Autodesk Inventor part; units mm, degrees
(part 2 of 3)
sketch "Sketch2" plane through (2, 0, 0) normal (1, 0, 0) x (0, 0, -1)
  line L0 (22.4898, 96.0981) -> (22.4898, 576.0981) projected
  line L1 (22.4898, 576.0981) -> (-367.5102, 576.0981) projected
  line L2 (-367.5102, 576.0981) -> (-367.5102, 96.0981) projected
  line L3 (-367.5102, 96.0981) -> (22.4898, 96.0981) projected
  circle A0 centre (-42.5102, 103.5981) radius 1.75 projected
  circle A1 centre (-302.5102, 568.5981) radius 1.75 projected
  circle A2 centre (-42.5102, 568.5981) radius 1.75 projected
  circle A3 centre (-360.0102, 161.0981) radius 1.75 projected
  circle A4 centre (-360.0102, 511.0981) radius 1.75 projected
  circle A5 centre (14.9898, 161.0981) radius 1.75 projected
  circle A6 centre (14.9898, 511.0981) radius 1.75 projected
  circle A7 centre (-172.5102, 568.5981) radius 1.75 projected
  circle A8 centre (-302.5102, 103.5981) radius 1.75 projected
  line L4 (2.265, 163.0981) -> (-3.5085, 163.0981) projected
  line L5 (-3.5085, 163.0981) -> (-6.3952, 168.0981) projected
  line L6 (-6.3952, 168.0981) -> (-3.5085, 173.0981) projected
  line L7 (-3.5085, 173.0981) -> (2.265, 173.0981) projected
  line L8 (2.265, 173.0981) -> (5.1518, 168.0981) projected
  line L9 (5.1518, 168.0981) -> (2.265, 163.0981) projected
  line L10 (-23.735, 143.0981) -> (-20.8482, 138.0981) projected
  line L11 (-20.8482, 138.0981) -> (-23.735, 133.0981) projected
  line L12 (-23.735, 133.0981) -> (-29.5085, 133.0981) projected
  line L13 (-29.5085, 133.0981) -> (-32.3952, 138.0981) projected
  line L14 (-32.3952, 138.0981) -> (-29.5085, 143.0981) projected
  line L15 (-29.5085, 143.0981) -> (-23.735, 143.0981) projected
  line L16 (-45.3856, 160.5981) -> (-42.4988, 165.5981) projected
  line L17 (-42.4988, 165.5981) -> (-36.7253, 165.5981) projected
  line L18 (-36.7253, 165.5981) -> (-33.8386, 160.5981) projected
  line L19 (-33.8386, 160.5981) -> (-36.7253, 155.5981) projected
  line L20 (-36.7253, 155.5981) -> (-42.4988, 155.5981) projected
  line L21 (-42.4988, 155.5981) -> (-45.3856, 160.5981) projected
  line L22 (-55.5085, 128.0981) -> (-49.735, 128.0981) projected
  line L23 (-49.735, 128.0981) -> (-46.8482, 123.0981) projected
  line L24 (-46.8482, 123.0981) -> (-49.735, 118.0981) projected
  line L25 (-49.735, 118.0981) -> (-55.5085, 118.0981) projected
  line L26 (-55.5085, 118.0981) -> (-58.3952, 123.0981) projected
  line L27 (-58.3952, 123.0981) -> (-55.5085, 128.0981) projected
  line L28 (-72.8482, 168.0981) -> (-75.735, 163.0981) projected
  line L29 (-75.735, 163.0981) -> (-81.5085, 163.0981) projected
  line L30 (-81.5085, 163.0981) -> (-84.3952, 168.0981) projected
  line L31 (-84.3952, 168.0981) -> (-81.5085, 173.0981) projected
  line L32 (-81.5085, 173.0981) -> (-75.735, 173.0981) projected
  line L33 (-75.735, 173.0981) -> (-72.8482, 168.0981) projected
  line L34 (-97.3856, 130.5981) -> (-94.4988, 135.5981) projected
  line L35 (-94.4988, 135.5981) -> (-88.7253, 135.5981) projected
  line L36 (-88.7253, 135.5981) -> (-85.8386, 130.5981) projected
  line L37 (-85.8386, 130.5981) -> (-88.7253, 125.5981) projected
  line L38 (-88.7253, 125.5981) -> (-94.4988, 125.5981) projected
  line L39 (-94.4988, 125.5981) -> (-97.3856, 130.5981) projected
  line L40 (-107.5085, 158.0981) -> (-101.735, 158.0981) projected
  line L41 (-101.735, 158.0981) -> (-98.8482, 153.0981) projected
  line L42 (-98.8482, 153.0981) -> (-101.735, 148.0981) projected
  line L43 (-101.735, 148.0981) -> (-107.5085, 148.0981) projected
  line L44 (-107.5085, 148.0981) -> (-110.3952, 153.0981) projected
  line L45 (-110.3952, 153.0981) -> (-107.5085, 158.0981) projected
  line L46 (-120.4988, 140.5981) -> (-123.3856, 145.5981) projected
  line L47 (-123.3856, 145.5981) -> (-120.4988, 150.5981) projected
  line L48 (-120.4988, 150.5981) -> (-114.7253, 150.5981) projected
  line L49 (-114.7253, 150.5981) -> (-111.8386, 145.5981) projected
  line L50 (-111.8386, 145.5981) -> (-114.7253, 140.5981) projected
  line L51 (-114.7253, 140.5981) -> (-120.4988, 140.5981) projected
  line L52 (-127.735, 143.0981) -> (-124.8482, 138.0981) projected
  line L53 (-124.8482, 138.0981) -> (-127.735, 133.0981) projected
  line L54 (-127.735, 133.0981) -> (-133.5085, 133.0981) projected
  line L55 (-133.5085, 133.0981) -> (-136.3952, 138.0981) projected
  line L56 (-136.3952, 138.0981) -> (-133.5085, 143.0981) projected
  line L57 (-133.5085, 143.0981) -> (-127.735, 143.0981) projected
  line L58 (-153.735, 143.0981) -> (-150.8482, 138.0981) projected
  line L59 (-150.8482, 138.0981) -> (-153.735, 133.0981) projected
  line L60 (-153.735, 133.0981) -> (-159.5085, 133.0981) projected
  line L61 (-159.5085, 133.0981) -> (-162.3952, 138.0981) projected
  line L62 (-162.3952, 138.0981) -> (-159.5085, 143.0981) projected
  line L63 (-159.5085, 143.0981) -> (-153.735, 143.0981) projected
  line L64 (-159.5085, 158.0981) -> (-153.735, 158.0981) projected
  line L65 (-153.735, 158.0981) -> (-150.8482, 153.0981) projected
  line L66 (-150.8482, 153.0981) -> (-153.735, 148.0981) projected
  line L67 (-153.735, 148.0981) -> (-159.5085, 148.0981) projected
  line L68 (-159.5085, 148.0981) -> (-162.3952, 153.0981) projected
  line L69 (-162.3952, 153.0981) -> (-159.5085, 158.0981) projected
  line L70 (-176.8482, 168.0981) -> (-179.735, 163.0981) projected
  line L71 (-179.735, 163.0981) -> (-185.5085, 163.0981) projected
  line L72 (-185.5085, 163.0981) -> (-188.3952, 168.0981) projected
  line L73 (-188.3952, 168.0981) -> (-185.5085, 173.0981) projected
  line L74 (-185.5085, 173.0981) -> (-179.735, 173.0981) projected
  line L75 (-179.735, 173.0981) -> (-176.8482, 168.0981) projected
  line L76 (-201.3856, 130.5981) -> (-198.4988, 135.5981) projected
  line L77 (-198.4988, 135.5981) -> (-192.7253, 135.5981) projected
  line L78 (-192.7253, 135.5981) -> (-189.8386, 130.5981) projected
  line L79 (-189.8386, 130.5981) -> (-192.7253, 125.5981) projected
  line L80 (-192.7253, 125.5981) -> (-198.4988, 125.5981) projected
  line L81 (-198.4988, 125.5981) -> (-201.3856, 130.5981) projected
  line L82 (-211.5085, 158.0981) -> (-205.735, 158.0981) projected
  line L83 (-205.735, 158.0981) -> (-202.8482, 153.0981) projected
  line L84 (-202.8482, 153.0981) -> (-205.735, 148.0981) projected
  line L85 (-205.735, 148.0981) -> (-211.5085, 148.0981) projected
  line L86 (-211.5085, 148.0981) -> (-214.3952, 153.0981) projected
  line L87 (-214.3952, 153.0981) -> (-211.5085, 158.0981) projected
  line L88 (-224.4988, 140.5981) -> (-227.3856, 145.5981) projected
  line L89 (-227.3856, 145.5981) -> (-224.4988, 150.5981) projected
  line L90 (-224.4988, 150.5981) -> (-218.7253, 150.5981) projected
  line L91 (-218.7253, 150.5981) -> (-215.8386, 145.5981) projected
  line L92 (-215.8386, 145.5981) -> (-218.7253, 140.5981) projected
  line L93 (-218.7253, 140.5981) -> (-224.4988, 140.5981) projected
  line L94 (-231.735, 143.0981) -> (-228.8482, 138.0981) projected
  line L95 (-228.8482, 138.0981) -> (-231.735, 133.0981) projected
  line L96 (-231.735, 133.0981) -> (-237.5085, 133.0981) projected
  line L97 (-237.5085, 133.0981) -> (-240.3952, 138.0981) projected
  line L98 (-240.3952, 138.0981) -> (-237.5085, 143.0981) projected
  line L99 (-237.5085, 143.0981) -> (-231.735, 143.0981) projected
  line L100 (-253.3856, 160.5981) -> (-250.4988, 165.5981) projected
  line L101 (-250.4988, 165.5981) -> (-244.7253, 165.5981) projected
  line L102 (-244.7253, 165.5981) -> (-241.8386, 160.5981) projected
  line L103 (-241.8386, 160.5981) -> (-244.7253, 155.5981) projected
  line L104 (-244.7253, 155.5981) -> (-250.4988, 155.5981) projected
  line L105 (-250.4988, 155.5981) -> (-253.3856, 160.5981) projected
  line L106 (-263.5085, 128.0981) -> (-257.735, 128.0981) projected
  line L107 (-257.735, 128.0981) -> (-254.8482, 123.0981) projected
  line L108 (-254.8482, 123.0981) -> (-257.735, 118.0981) projected
  line L109 (-257.735, 118.0981) -> (-263.5085, 118.0981) projected
  line L110 (-263.5085, 118.0981) -> (-266.3952, 123.0981) projected
  line L111 (-266.3952, 123.0981) -> (-263.5085, 128.0981) projected
  line L112 (-315.5085, 128.0981) -> (-309.735, 128.0981) projected
  line L113 (-309.735, 128.0981) -> (-306.8482, 123.0981) projected
  line L114 (-306.8482, 123.0981) -> (-309.735, 118.0981) projected
  line L115 (-309.735, 118.0981) -> (-315.5085, 118.0981) projected
  line L116 (-315.5085, 118.0981) -> (-318.3952, 123.0981) projected
  line L117 (-318.3952, 123.0981) -> (-315.5085, 128.0981) projected
  line L118 (-341.5085, 158.0981) -> (-335.735, 158.0981) projected
  line L119 (-335.735, 158.0981) -> (-332.8482, 153.0981) projected
  line L120 (-332.8482, 153.0981) -> (-335.735, 148.0981) projected
  line L121 (-335.735, 148.0981) -> (-341.5085, 148.0981) projected
  line L122 (-341.5085, 148.0981) -> (-344.3952, 153.0981) projected
  line L123 (-344.3952, 153.0981) -> (-341.5085, 158.0981) projected
  line L124 (-280.8482, 168.0981) -> (-283.735, 163.0981) projected
  line L125 (-283.735, 163.0981) -> (-289.5085, 163.0981) projected
  line L126 (-289.5085, 163.0981) -> (-292.3952, 168.0981) projected
  line L127 (-292.3952, 168.0981) -> (-289.5085, 173.0981) projected
  line L128 (-289.5085, 173.0981) -> (-283.735, 173.0981) projected
  line L129 (-283.735, 173.0981) -> (-280.8482, 168.0981) projected
  line L130 (-283.735, 143.0981) -> (-280.8482, 138.0981) projected
  line L131 (-280.8482, 138.0981) -> (-283.735, 133.0981) projected
  line L132 (-283.735, 133.0981) -> (-289.5085, 133.0981) projected
  line L133 (-289.5085, 133.0981) -> (-292.3952, 138.0981) projected
  line L134 (-292.3952, 138.0981) -> (-289.5085, 143.0981) projected
  line L135 (-289.5085, 143.0981) -> (-283.735, 143.0981) projected
  line L136 (-309.735, 143.0981) -> (-306.8482, 138.0981) projected
  line L137 (-306.8482, 138.0981) -> (-309.735, 133.0981) projected
  line L138 (-309.735, 133.0981) -> (-315.5085, 133.0981) projected
  line L139 (-315.5085, 133.0981) -> (-318.3952, 138.0981) projected
  line L140 (-318.3952, 138.0981) -> (-315.5085, 143.0981) projected
  line L141 (-315.5085, 143.0981) -> (-309.735, 143.0981) projected
  line L142 (-3.5085, 128.0981) -> (2.265, 128.0981) projected
  line L143 (2.265, 128.0981) -> (5.1518, 123.0981) projected
  line L144 (5.1518, 123.0981) -> (2.265, 118.0981) projected
  line L145 (2.265, 118.0981) -> (-3.5085, 118.0981) projected
  line L146 (-3.5085, 118.0981) -> (-6.3952, 123.0981) projected
  line L147 (-6.3952, 123.0981) -> (-3.5085, 128.0981) projected
  line L148 (-10.7253, 140.5981) -> (-16.4988, 140.5981) projected
  line L149 (-16.4988, 140.5981) -> (-19.3856, 145.5981) projected
  line L150 (-19.3856, 145.5981) -> (-16.4988, 150.5981) projected
  line L151 (-16.4988, 150.5981) -> (-10.7253, 150.5981) projected
  line L152 (-10.7253, 150.5981) -> (-7.8386, 145.5981) projected
  line L153 (-7.8386, 145.5981) -> (-10.7253, 140.5981) projected
  line L154 (-328.4988, 140.5981) -> (-331.3856, 145.5981) projected
  line L155 (-331.3856, 145.5981) -> (-328.4988, 150.5981) projected
  line L156 (-328.4988, 150.5981) -> (-322.7253, 150.5981) projected
  line L157 (-322.7253, 150.5981) -> (-319.8386, 145.5981) projected
  line L158 (-319.8386, 145.5981) -> (-322.7253, 140.5981) projected
  line L159 (-322.7253, 140.5981) -> (-328.4988, 140.5981) projected
  line L160 (-302.4988, 140.5981) -> (-305.3856, 145.5981) projected
  line L161 (-305.3856, 145.5981) -> (-302.4988, 150.5981) projected
  line L162 (-302.4988, 150.5981) -> (-296.7253, 150.5981) projected
  line L163 (-296.7253, 150.5981) -> (-293.8386, 145.5981) projected
  line L164 (-293.8386, 145.5981) -> (-296.7253, 140.5981) projected
  line L165 (-296.7253, 140.5981) -> (-302.4988, 140.5981) projected
  line L166 (-279.3856, 160.5981) -> (-276.4988, 165.5981) projected
  line L167 (-276.4988, 165.5981) -> (-270.7253, 165.5981) projected
  line L168 (-270.7253, 165.5981) -> (-267.8386, 160.5981) projected
  line L169 (-267.8386, 160.5981) -> (-270.7253, 155.5981) projected
  line L170 (-270.7253, 155.5981) -> (-276.4988, 155.5981) projected
  line L171 (-276.4988, 155.5981) -> (-279.3856, 160.5981) projected
  line L172 (-332.8482, 168.0981) -> (-335.735, 163.0981) projected
  line L173 (-335.735, 163.0981) -> (-341.5085, 163.0981) projected
  line L174 (-341.5085, 163.0981) -> (-344.3952, 168.0981) projected
  line L175 (-344.3952, 168.0981) -> (-341.5085, 173.0981) projected
  line L176 (-341.5085, 173.0981) -> (-335.735, 173.0981) projected
  line L177 (-335.735, 173.0981) -> (-332.8482, 168.0981) projected
  line L178 (-331.3856, 130.5981) -> (-328.4988, 135.5981) projected
  line L179 (-328.4988, 135.5981) -> (-322.7253, 135.5981) projected
  line L180 (-322.7253, 135.5981) -> (-319.8386, 130.5981) projected
  line L181 (-319.8386, 130.5981) -> (-322.7253, 125.5981) projected
  line L182 (-322.7253, 125.5981) -> (-328.4988, 125.5981) projected
  line L183 (-328.4988, 125.5981) -> (-331.3856, 130.5981) projected
  line L184 (-279.3856, 130.5981) -> (-276.4988, 135.5981) projected
  line L185 (-276.4988, 135.5981) -> (-270.7253, 135.5981) projected
  line L186 (-270.7253, 135.5981) -> (-267.8386, 130.5981) projected
  line L187 (-267.8386, 130.5981) -> (-270.7253, 125.5981) projected
  line L188 (-270.7253, 125.5981) -> (-276.4988, 125.5981) projected
  line L189 (-276.4988, 125.5981) -> (-279.3856, 130.5981) projected
  line L190 (-254.8482, 168.0981) -> (-257.735, 163.0981) projected
  line L191 (-257.735, 163.0981) -> (-263.5085, 163.0981) projected
  line L192 (-263.5085, 163.0981) -> (-266.3952, 168.0981) projected
  line L193 (-266.3952, 168.0981) -> (-263.5085, 173.0981) projected
  line L194 (-263.5085, 173.0981) -> (-257.735, 173.0981) projected
  line L195 (-257.735, 173.0981) -> (-254.8482, 168.0981) projected
  line L196 (-237.5085, 128.0981) -> (-231.735, 128.0981) projected
  line L197 (-231.735, 128.0981) -> (-228.8482, 123.0981) projected
  line L198 (-228.8482, 123.0981) -> (-231.735, 118.0981) projected
  line L199 (-231.735, 118.0981) -> (-237.5085, 118.0981) projected
  line L200 (-237.5085, 118.0981) -> (-240.3952, 123.0981) projected
  line L201 (-240.3952, 123.0981) -> (-237.5085, 128.0981) projected
  line L202 (-227.3856, 160.5981) -> (-224.4988, 165.5981) projected
  line L203 (-224.4988, 165.5981) -> (-218.7253, 165.5981) projected
  line L204 (-218.7253, 165.5981) -> (-215.8386, 160.5981) projected
  line L205 (-215.8386, 160.5981) -> (-218.7253, 155.5981) projected
  line L206 (-218.7253, 155.5981) -> (-224.4988, 155.5981) projected
  line L207 (-224.4988, 155.5981) -> (-227.3856, 160.5981) projected
  line L208 (-205.735, 143.0981) -> (-202.8482, 138.0981) projected
  line L209 (-202.8482, 138.0981) -> (-205.735, 133.0981) projected
  line L210 (-205.735, 133.0981) -> (-211.5085, 133.0981) projected
  line L211 (-211.5085, 133.0981) -> (-214.3952, 138.0981) projected
  line L212 (-214.3952, 138.0981) -> (-211.5085, 143.0981) projected
  line L213 (-211.5085, 143.0981) -> (-205.735, 143.0981) projected
  line L214 (-198.4988, 140.5981) -> (-201.3856, 145.5981) projected
  line L215 (-201.3856, 145.5981) -> (-198.4988, 150.5981) projected
  line L216 (-198.4988, 150.5981) -> (-192.7253, 150.5981) projected
  line L217 (-192.7253, 150.5981) -> (-189.8386, 145.5981) projected
  line L218 (-189.8386, 145.5981) -> (-192.7253, 140.5981) projected
  line L219 (-192.7253, 140.5981) -> (-198.4988, 140.5981) projected
  line L220 (-185.5085, 158.0981) -> (-179.735, 158.0981) projected
  line L221 (-179.735, 158.0981) -> (-176.8482, 153.0981) projected
  line L222 (-176.8482, 153.0981) -> (-179.735, 148.0981) projected
  line L223 (-179.735, 148.0981) -> (-185.5085, 148.0981) projected
  line L224 (-185.5085, 148.0981) -> (-188.3952, 153.0981) projected
  line L225 (-188.3952, 153.0981) -> (-185.5085, 158.0981) projected
  line L226 (-175.3856, 130.5981) -> (-172.4988, 135.5981) projected
  line L227 (-172.4988, 135.5981) -> (-166.7253, 135.5981) projected
  line L228 (-166.7253, 135.5981) -> (-163.8386, 130.5981) projected
  line L229 (-163.8386, 130.5981) -> (-166.7253, 125.5981) projected
  line L230 (-166.7253, 125.5981) -> (-172.4988, 125.5981) projected
  line L231 (-172.4988, 125.5981) -> (-175.3856, 130.5981) projected
  line L232 (-146.4988, 140.5981) -> (-149.3856, 145.5981) projected
  line L233 (-149.3856, 145.5981) -> (-146.4988, 150.5981) projected
  line L234 (-146.4988, 150.5981) -> (-140.7253, 150.5981) projected
  line L235 (-140.7253, 150.5981) -> (-137.8386, 145.5981) projected
  line L236 (-137.8386, 145.5981) -> (-140.7253, 140.5981) projected
  line L237 (-140.7253, 140.5981) -> (-146.4988, 140.5981) projected
  line L238 (-133.5085, 128.0981) -> (-127.735, 128.0981) projected
  line L239 (-127.735, 128.0981) -> (-124.8482, 123.0981) projected
  line L240 (-124.8482, 123.0981) -> (-127.735, 118.0981) projected
  line L241 (-127.735, 118.0981) -> (-133.5085, 118.0981) projected
  line L242 (-133.5085, 118.0981) -> (-136.3952, 123.0981) projected
  line L243 (-136.3952, 123.0981) -> (-133.5085, 128.0981) projected
  line L244 (-123.3856, 160.5981) -> (-120.4988, 165.5981) projected
  line L245 (-120.4988, 165.5981) -> (-114.7253, 165.5981) projected
  line L246 (-114.7253, 165.5981) -> (-111.8386, 160.5981) projected
  line L247 (-111.8386, 160.5981) -> (-114.7253, 155.5981) projected
  line L248 (-114.7253, 155.5981) -> (-120.4988, 155.5981) projected
  line L249 (-120.4988, 155.5981) -> (-123.3856, 160.5981) projected
  line L250 (-101.735, 143.0981) -> (-98.8482, 138.0981) projected
  line L251 (-98.8482, 138.0981) -> (-101.735, 133.0981) projected
  line L252 (-101.735, 133.0981) -> (-107.5085, 133.0981) projected
  line L253 (-107.5085, 133.0981) -> (-110.3952, 138.0981) projected
  line L254 (-110.3952, 138.0981) -> (-107.5085, 143.0981) projected
  line L255 (-107.5085, 143.0981) -> (-101.735, 143.0981) projected
  line L256 (-94.4988, 140.5981) -> (-97.3856, 145.5981) projected
  line L257 (-97.3856, 145.5981) -> (-94.4988, 150.5981) projected
  line L258 (-94.4988, 150.5981) -> (-88.7253, 150.5981) projected
  line L259 (-88.7253, 150.5981) -> (-85.8386, 145.5981) projected
  line L260 (-85.8386, 145.5981) -> (-88.7253, 140.5981) projected
  line L261 (-88.7253, 140.5981) -> (-94.4988, 140.5981) projected
  line L262 (-81.5085, 158.0981) -> (-75.735, 158.0981) projected
  line L263 (-75.735, 158.0981) -> (-72.8482, 153.0981) projected
  line L264 (-72.8482, 153.0981) -> (-75.735, 148.0981) projected
  line L265 (-75.735, 148.0981) -> (-81.5085, 148.0981) projected
  line L266 (-81.5085, 148.0981) -> (-84.3952, 153.0981) projected
  line L267 (-84.3952, 153.0981) -> (-81.5085, 158.0981) projected
  line L268 (-71.3856, 130.5981) -> (-68.4988, 135.5981) projected
  line L269 (-68.4988, 135.5981) -> (-62.7253, 135.5981) projected
  line L270 (-62.7253, 135.5981) -> (-59.8386, 130.5981) projected
  line L271 (-59.8386, 130.5981) -> (-62.7253, 125.5981) projected
  line L272 (-62.7253, 125.5981) -> (-68.4988, 125.5981) projected
  line L273 (-68.4988, 125.5981) -> (-71.3856, 130.5981) projected
  line L274 (-46.8482, 168.0981) -> (-49.735, 163.0981) projected
  line L275 (-49.735, 163.0981) -> (-55.5085, 163.0981) projected
  line L276 (-55.5085, 163.0981) -> (-58.3952, 168.0981) projected
  line L277 (-58.3952, 168.0981) -> (-55.5085, 173.0981) projected
  line L278 (-55.5085, 173.0981) -> (-49.735, 173.0981) projected
  line L279 (-49.735, 173.0981) -> (-46.8482, 168.0981) projected
  line L280 (-29.5085, 128.0981) -> (-23.735, 128.0981) projected
  line L281 (-23.735, 128.0981) -> (-20.8482, 123.0981) projected
  line L282 (-20.8482, 123.0981) -> (-23.735, 118.0981) projected
  line L283 (-23.735, 118.0981) -> (-29.5085, 118.0981) projected
  line L284 (-29.5085, 118.0981) -> (-32.3952, 123.0981) projected
  line L285 (-32.3952, 123.0981) -> (-29.5085, 128.0981) projected
  line L286 (-10.7253, 155.5981) -> (-16.4988, 155.5981) projected
  line L287 (-16.4988, 155.5981) -> (-19.3856, 160.5981) projected
  line L288 (-19.3856, 160.5981) -> (-16.4988, 165.5981) projected
  line L289 (-16.4988, 165.5981) -> (-10.7253, 165.5981) projected
  line L290 (-10.7253, 165.5981) -> (-7.8386, 160.5981) projected
  line L291 (-7.8386, 160.5981) -> (-10.7253, 155.5981) projected
  line L292 (-29.5085, 158.0981) -> (-23.735, 158.0981) projected
  line L293 (-23.735, 158.0981) -> (-20.8482, 153.0981) projected
  line L294 (-20.8482, 153.0981) -> (-23.735, 148.0981) projected
  line L295 (-23.735, 148.0981) -> (-29.5085, 148.0981) projected
  line L296 (-29.5085, 148.0981) -> (-32.3952, 153.0981) projected
  line L297 (-32.3952, 153.0981) -> (-29.5085, 158.0981) projected
  line L298 (-42.4988, 140.5981) -> (-45.3856, 145.5981) projected
  line L299 (-45.3856, 145.5981) -> (-42.4988, 150.5981) projected
  line L300 (-42.4988, 150.5981) -> (-36.7253, 150.5981) projected
  line L301 (-36.7253, 150.5981) -> (-33.8386, 145.5981) projected
  line L302 (-33.8386, 145.5981) -> (-36.7253, 140.5981) projected
  line L303 (-36.7253, 140.5981) -> (-42.4988, 140.5981) projected
  line L304 (-49.735, 143.0981) -> (-46.8482, 138.0981) projected
  line L305 (-46.8482, 138.0981) -> (-49.735, 133.0981) projected
  line L306 (-49.735, 133.0981) -> (-55.5085, 133.0981) projected
  line L307 (-55.5085, 133.0981) -> (-58.3952, 138.0981) projected
  line L308 (-58.3952, 138.0981) -> (-55.5085, 143.0981) projected
  line L309 (-55.5085, 143.0981) -> (-49.735, 143.0981) projected
  line L310 (-71.3856, 160.5981) -> (-68.4988, 165.5981) projected
  line L311 (-68.4988, 165.5981) -> (-62.7253, 165.5981) projected
  line L312 (-62.7253, 165.5981) -> (-59.8386, 160.5981) projected
  line L313 (-59.8386, 160.5981) -> (-62.7253, 155.5981) projected
  line L314 (-62.7253, 155.5981) -> (-68.4988, 155.5981) projected
  line L315 (-68.4988, 155.5981) -> (-71.3856, 160.5981) projected
  line L316 (-81.5085, 128.0981) -> (-75.735, 128.0981) projected
  line L317 (-75.735, 128.0981) -> (-72.8482, 123.0981) projected
  line L318 (-72.8482, 123.0981) -> (-75.735, 118.0981) projected
  line L319 (-75.735, 118.0981) -> (-81.5085, 118.0981) projected
  line L320 (-81.5085, 118.0981) -> (-84.3952, 123.0981) projected
  line L321 (-84.3952, 123.0981) -> (-81.5085, 128.0981) projected
  line L322 (-98.8482, 168.0981) -> (-101.735, 163.0981) projected
  line L323 (-101.735, 163.0981) -> (-107.5085, 163.0981) projected
  line L324 (-107.5085, 163.0981) -> (-110.3952, 168.0981) projected
  line L325 (-110.3952, 168.0981) -> (-107.5085, 173.0981) projected
  line L326 (-107.5085, 173.0981) -> (-101.735, 173.0981) projected
  line L327 (-101.735, 173.0981) -> (-98.8482, 168.0981) projected
  line L328 (-123.3856, 130.5981) -> (-120.4988, 135.5981) projected
  line L329 (-120.4988, 135.5981) -> (-114.7253, 135.5981) projected
  line L330 (-114.7253, 135.5981) -> (-111.8386, 130.5981) projected
  line L331 (-111.8386, 130.5981) -> (-114.7253, 125.5981) projected
  line L332 (-114.7253, 125.5981) -> (-120.4988, 125.5981) projected
  line L333 (-120.4988, 125.5981) -> (-123.3856, 130.5981) projected
  line L334 (-133.5085, 158.0981) -> (-127.735, 158.0981) projected
  line L335 (-127.735, 158.0981) -> (-124.8482, 153.0981) projected
  line L336 (-124.8482, 153.0981) -> (-127.735, 148.0981) projected
  line L337 (-127.735, 148.0981) -> (-133.5085, 148.0981) projected
  line L338 (-133.5085, 148.0981) -> (-136.3952, 153.0981) projected
  line L339 (-136.3952, 153.0981) -> (-133.5085, 158.0981) projected
  line L340 (-159.5085, 128.0981) -> (-153.735, 128.0981) projected
  line L341 (-153.735, 128.0981) -> (-150.8482, 123.0981) projected
  line L342 (-150.8482, 123.0981) -> (-153.735, 118.0981) projected
  line L343 (-153.735, 118.0981) -> (-159.5085, 118.0981) projected
  line L344 (-159.5085, 118.0981) -> (-162.3952, 123.0981) projected
  line L345 (-162.3952, 123.0981) -> (-159.5085, 128.0981) projected
  line L346 (-150.8482, 168.0981) -> (-153.735, 163.0981) projected
  line L347 (-153.735, 163.0981) -> (-159.5085, 163.0981) projected
  line L348 (-159.5085, 163.0981) -> (-162.3952, 168.0981) projected
  line L349 (-162.3952, 168.0981) -> (-159.5085, 173.0981) projected
  line L350 (-159.5085, 173.0981) -> (-153.735, 173.0981) projected
  line L351 (-153.735, 173.0981) -> (-150.8482, 168.0981) projected
  line L352 (-175.3856, 160.5981) -> (-172.4988, 165.5981) projected
  line L353 (-172.4988, 165.5981) -> (-166.7253, 165.5981) projected
  line L354 (-166.7253, 165.5981) -> (-163.8386, 160.5981) projected
  line L355 (-163.8386, 160.5981) -> (-166.7253, 155.5981) projected
  line L356 (-166.7253, 155.5981) -> (-172.4988, 155.5981) projected
  line L357 (-172.4988, 155.5981) -> (-175.3856, 160.5981) projected
  line L358 (-185.5085, 128.0981) -> (-179.735, 128.0981) projected
  line L359 (-179.735, 128.0981) -> (-176.8482, 123.0981) projected
  line L360 (-176.8482, 123.0981) -> (-179.735, 118.0981) projected
  line L361 (-179.735, 118.0981) -> (-185.5085, 118.0981) projected
  line L362 (-185.5085, 118.0981) -> (-188.3952, 123.0981) projected
  line L363 (-188.3952, 123.0981) -> (-185.5085, 128.0981) projected
  line L364 (-202.8482, 168.0981) -> (-205.735, 163.0981) projected
  line L365 (-205.735, 163.0981) -> (-211.5085, 163.0981) projected
  line L366 (-211.5085, 163.0981) -> (-214.3952, 168.0981) projected
  line L367 (-214.3952, 168.0981) -> (-211.5085, 173.0981) projected
  line L368 (-211.5085, 173.0981) -> (-205.735, 173.0981) projected
  line L369 (-205.735, 173.0981) -> (-202.8482, 168.0981) projected
  line L370 (-227.3856, 130.5981) -> (-224.4988, 135.5981) projected
  line L371 (-224.4988, 135.5981) -> (-218.7253, 135.5981) projected
  line L372 (-218.7253, 135.5981) -> (-215.8386, 130.5981) projected
  line L373 (-215.8386, 130.5981) -> (-218.7253, 125.5981) projected
  line L374 (-218.7253, 125.5981) -> (-224.4988, 125.5981) projected
  line L375 (-224.4988, 125.5981) -> (-227.3856, 130.5981) projected
  line L376 (-237.5085, 158.0981) -> (-231.735, 158.0981) projected
  line L377 (-231.735, 158.0981) -> (-228.8482, 153.0981) projected
  line L378 (-228.8482, 153.0981) -> (-231.735, 148.0981) projected
  line L379 (-231.735, 148.0981) -> (-237.5085, 148.0981) projected
  line L380 (-237.5085, 148.0981) -> (-240.3952, 153.0981) projected
  line L381 (-240.3952, 153.0981) -> (-237.5085, 158.0981) projected
  line L382 (-250.4988, 140.5981) -> (-253.3856, 145.5981) projected
  line L383 (-253.3856, 145.5981) -> (-250.4988, 150.5981) projected
  line L384 (-250.4988, 150.5981) -> (-244.7253, 150.5981) projected
  line L385 (-244.7253, 150.5981) -> (-241.8386, 145.5981) projected
  line L386 (-241.8386, 145.5981) -> (-244.7253, 140.5981) projected
  line L387 (-244.7253, 140.5981) -> (-250.4988, 140.5981) projected
  line L388 (-257.735, 143.0981) -> (-254.8482, 138.0981) projected
  line L389 (-254.8482, 138.0981) -> (-257.735, 133.0981) projected
  line L390 (-257.735, 133.0981) -> (-263.5085, 133.0981) projected
  line L391 (-263.5085, 133.0981) -> (-266.3952, 138.0981) projected
  line L392 (-266.3952, 138.0981) -> (-263.5085, 143.0981) projected
  line L393 (-263.5085, 143.0981) -> (-257.735, 143.0981) projected
  line L394 (-305.3856, 130.5981) -> (-302.4988, 135.5981) projected
  line L395 (-302.4988, 135.5981) -> (-296.7253, 135.5981) projected
  line L396 (-296.7253, 135.5981) -> (-293.8386, 130.5981) projected
  line L397 (-293.8386, 130.5981) -> (-296.7253, 125.5981) projected
  line L398 (-296.7253, 125.5981) -> (-302.4988, 125.5981) projected
  line L399 (-302.4988, 125.5981) -> (-305.3856, 130.5981) projected
  line L400 (-335.735, 143.0981) -> (-332.8482, 138.0981) projected
  line L401 (-332.8482, 138.0981) -> (-335.735, 133.0981) projected
  line L402 (-335.735, 133.0981) -> (-341.5085, 133.0981) projected
  line L403 (-341.5085, 133.0981) -> (-344.3952, 138.0981) projected
  line L404 (-344.3952, 138.0981) -> (-341.5085, 143.0981) projected
  line L405 (-341.5085, 143.0981) -> (-335.735, 143.0981) projected
  line L406 (-306.8482, 168.0981) -> (-309.735, 163.0981) projected
  line L407 (-309.735, 163.0981) -> (-315.5085, 163.0981) projected
  line L408 (-315.5085, 163.0981) -> (-318.3952, 168.0981) projected
  line L409 (-318.3952, 168.0981) -> (-315.5085, 173.0981) projected
  line L410 (-315.5085, 173.0981) -> (-309.735, 173.0981) projected
  line L411 (-309.735, 173.0981) -> (-306.8482, 168.0981) projected
  line L412 (-289.5085, 158.0981) -> (-283.735, 158.0981) projected
  line L413 (-283.735, 158.0981) -> (-280.8482, 153.0981) projected
  line L414 (-280.8482, 153.0981) -> (-283.735, 148.0981) projected
  line L415 (-283.735, 148.0981) -> (-289.5085, 148.0981) projected
  line L416 (-289.5085, 148.0981) -> (-292.3952, 153.0981) projected
  line L417 (-292.3952, 153.0981) -> (-289.5085, 158.0981) projected
  line L418 (-315.5085, 158.0981) -> (-309.735, 158.0981) projected
  line L419 (-309.735, 158.0981) -> (-306.8482, 153.0981) projected
  line L420 (-306.8482, 153.0981) -> (-309.735, 148.0981) projected
  line L421 (-309.735, 148.0981) -> (-315.5085, 148.0981) projected
  line L422 (-315.5085, 148.0981) -> (-318.3952, 153.0981) projected
  line L423 (-318.3952, 153.0981) -> (-315.5085, 158.0981) projected
  line L424 (2.265, 148.0981) -> (-3.5085, 148.0981) projected
  line L425 (-3.5085, 148.0981) -> (-6.3952, 153.0981) projected
  line L426 (-6.3952, 153.0981) -> (-3.5085, 158.0981) projected
  line L427 (-3.5085, 158.0981) -> (2.265, 158.0981) projected
  line L428 (2.265, 158.0981) -> (5.1518, 153.0981) projected
  line L429 (5.1518, 153.0981) -> (2.265, 148.0981) projected
  line L430 (-19.3856, 130.5981) -> (-16.4988, 135.5981) projected
  line L431 (-16.4988, 135.5981) -> (-10.7253, 135.5981) projected
  line L432 (-10.7253, 135.5981) -> (-7.8386, 130.5981) projected
  line L433 (-7.8386, 130.5981) -> (-10.7253, 125.5981) projected
  line L434 (-10.7253, 125.5981) -> (-16.4988, 125.5981) projected
  line L435 (-16.4988, 125.5981) -> (-19.3856, 130.5981) projected
  line L436 (-3.5085, 143.0981) -> (2.265, 143.0981) projected
  line L437 (2.265, 143.0981) -> (5.1518, 138.0981) projected
  line L438 (5.1518, 138.0981) -> (2.265, 133.0981) projected
  line L439 (2.265, 133.0981) -> (-3.5085, 133.0981) projected
  line L440 (-3.5085, 133.0981) -> (-6.3952, 138.0981) projected
  line L441 (-6.3952, 138.0981) -> (-3.5085, 143.0981) projected
  line L442 (-305.3856, 160.5981) -> (-302.4988, 165.5981) projected
  line L443 (-302.4988, 165.5981) -> (-296.7253, 165.5981) projected
  line L444 (-296.7253, 165.5981) -> (-293.8386, 160.5981) projected
  line L445 (-293.8386, 160.5981) -> (-296.7253, 155.5981) projected
  line L446 (-296.7253, 155.5981) -> (-302.4988, 155.5981) projected
  line L447 (-302.4988, 155.5981) -> (-305.3856, 160.5981) projected
  line L448 (-276.4988, 140.5981) -> (-279.3856, 145.5981) projected
  line L449 (-279.3856, 145.5981) -> (-276.4988, 150.5981) projected
  line L450 (-276.4988, 150.5981) -> (-270.7253, 150.5981) projected
  line L451 (-270.7253, 150.5981) -> (-267.8386, 145.5981) projected
  line L452 (-267.8386, 145.5981) -> (-270.7253, 140.5981) projected
  line L453 (-270.7253, 140.5981) -> (-276.4988, 140.5981) projected
  line L454 (-331.3856, 160.5981) -> (-328.4988, 165.5981) projected
  line L455 (-328.4988, 165.5981) -> (-322.7253, 165.5981) projected
  line L456 (-322.7253, 165.5981) -> (-319.8386, 160.5981) projected
  line L457 (-319.8386, 160.5981) -> (-322.7253, 155.5981) projected
  line L458 (-322.7253, 155.5981) -> (-328.4988, 155.5981) projected
  line L459 (-328.4988, 155.5981) -> (-331.3856, 160.5981) projected
  line L460 (-341.5085, 128.0981) -> (-335.735, 128.0981) projected
  line L461 (-335.735, 128.0981) -> (-332.8482, 123.0981) projected
  line L462 (-332.8482, 123.0981) -> (-335.735, 118.0981) projected
  line L463 (-335.735, 118.0981) -> (-341.5085, 118.0981) projected
  line L464 (-341.5085, 118.0981) -> (-344.3952, 123.0981) projected
  line L465 (-344.3952, 123.0981) -> (-341.5085, 128.0981) projected
  line L466 (-289.5085, 128.0981) -> (-283.735, 128.0981) projected
  line L467 (-283.735, 128.0981) -> (-280.8482, 123.0981) projected
  line L468 (-280.8482, 123.0981) -> (-283.735, 118.0981) projected
  line L469 (-283.735, 118.0981) -> (-289.5085, 118.0981) projected
  line L470 (-289.5085, 118.0981) -> (-292.3952, 123.0981) projected
  line L471 (-292.3952, 123.0981) -> (-289.5085, 128.0981) projected
  line L472 (-263.5085, 158.0981) -> (-257.735, 158.0981) projected
  line L473 (-257.735, 158.0981) -> (-254.8482, 153.0981) projected
  line L474 (-254.8482, 153.0981) -> (-257.735, 148.0981) projected
  line L475 (-257.735, 148.0981) -> (-263.5085, 148.0981) projected
  line L476 (-263.5085, 148.0981) -> (-266.3952, 153.0981) projected
  line L477 (-266.3952, 153.0981) -> (-263.5085, 158.0981) projected
  line L478 (-253.3856, 130.5981) -> (-250.4988, 135.5981) projected
  line L479 (-250.4988, 135.5981) -> (-244.7253, 135.5981) projected
  line L480 (-244.7253, 135.5981) -> (-241.8386, 130.5981) projected
  line L481 (-241.8386, 130.5981) -> (-244.7253, 125.5981) projected
  line L482 (-244.7253, 125.5981) -> (-250.4988, 125.5981) projected
  line L483 (-250.4988, 125.5981) -> (-253.3856, 130.5981) projected
  line L484 (-228.8482, 168.0981) -> (-231.735, 163.0981) projected
  line L485 (-231.735, 163.0981) -> (-237.5085, 163.0981) projected
  line L486 (-237.5085, 163.0981) -> (-240.3952, 168.0981) projected
  line L487 (-240.3952, 168.0981) -> (-237.5085, 173.0981) projected
  line L488 (-237.5085, 173.0981) -> (-231.735, 173.0981) projected
  line L489 (-231.735, 173.0981) -> (-228.8482, 168.0981) projected
  line L490 (-211.5085, 128.0981) -> (-205.735, 128.0981) projected
  line L491 (-205.735, 128.0981) -> (-202.8482, 123.0981) projected
  line L492 (-202.8482, 123.0981) -> (-205.735, 118.0981) projected
  line L493 (-205.735, 118.0981) -> (-211.5085, 118.0981) projected
  line L494 (-211.5085, 118.0981) -> (-214.3952, 123.0981) projected
  line L495 (-214.3952, 123.0981) -> (-211.5085, 128.0981) projected
  line L496 (-201.3856, 160.5981) -> (-198.4988, 165.5981) projected
  line L497 (-198.4988, 165.5981) -> (-192.7253, 165.5981) projected
  line L498 (-192.7253, 165.5981) -> (-189.8386, 160.5981) projected
  line L499 (-189.8386, 160.5981) -> (-192.7253, 155.5981) projected
  line L500 (-192.7253, 155.5981) -> (-198.4988, 155.5981) projected
  line L501 (-198.4988, 155.5981) -> (-201.3856, 160.5981) projected
  line L502 (-179.735, 143.0981) -> (-176.8482, 138.0981) projected
  line L503 (-176.8482, 138.0981) -> (-179.735, 133.0981) projected
  line L504 (-179.735, 133.0981) -> (-185.5085, 133.0981) projected
  line L505 (-185.5085, 133.0981) -> (-188.3952, 138.0981) projected
  line L506 (-188.3952, 138.0981) -> (-185.5085, 143.0981) projected
  line L507 (-185.5085, 143.0981) -> (-179.735, 143.0981) projected
  line L508 (-172.4988, 140.5981) -> (-175.3856, 145.5981) projected
  line L509 (-175.3856, 145.5981) -> (-172.4988, 150.5981) projected
  line L510 (-172.4988, 150.5981) -> (-166.7253, 150.5981) projected
  line L511 (-166.7253, 150.5981) -> (-163.8386, 145.5981) projected
  line L512 (-163.8386, 145.5981) -> (-166.7253, 140.5981) projected
  line L513 (-166.7253, 140.5981) -> (-172.4988, 140.5981) projected
  line L514 (-149.3856, 160.5981) -> (-146.4988, 165.5981) projected
  line L515 (-146.4988, 165.5981) -> (-140.7253, 165.5981) projected
  line L516 (-140.7253, 165.5981) -> (-137.8386, 160.5981) projected
  line L517 (-137.8386, 160.5981) -> (-140.7253, 155.5981) projected
  line L518 (-140.7253, 155.5981) -> (-146.4988, 155.5981) projected
  line L519 (-146.4988, 155.5981) -> (-149.3856, 160.5981) projected
  line L520 (-149.3856, 130.5981) -> (-146.4988, 135.5981) projected
  line L521 (-146.4988, 135.5981) -> (-140.7253, 135.5981) projected
  line L522 (-140.7253, 135.5981) -> (-137.8386, 130.5981) projected
  line L523 (-137.8386, 130.5981) -> (-140.7253, 125.5981) projected
  line L524 (-140.7253, 125.5981) -> (-146.4988, 125.5981) projected
  line L525 (-146.4988, 125.5981) -> (-149.3856, 130.5981) projected
  line L526 (-124.8482, 168.0981) -> (-127.735, 163.0981) projected
  line L527 (-127.735, 163.0981) -> (-133.5085, 163.0981) projected
  line L528 (-133.5085, 163.0981) -> (-136.3952, 168.0981) projected
  line L529 (-136.3952, 168.0981) -> (-133.5085, 173.0981) projected
  line L530 (-133.5085, 173.0981) -> (-127.735, 173.0981) projected
  line L531 (-127.735, 173.0981) -> (-124.8482, 168.0981) projected
  line L532 (-107.5085, 128.0981) -> (-101.735, 128.0981) projected
  line L533 (-101.735, 128.0981) -> (-98.8482, 123.0981) projected
  line L534 (-98.8482, 123.0981) -> (-101.735, 118.0981) projected
  line L535 (-101.735, 118.0981) -> (-107.5085, 118.0981) projected
  line L536 (-107.5085, 118.0981) -> (-110.3952, 123.0981) projected
  line L537 (-110.3952, 123.0981) -> (-107.5085, 128.0981) projected
  line L538 (-97.3856, 160.5981) -> (-94.4988, 165.5981) projected
  line L539 (-94.4988, 165.5981) -> (-88.7253, 165.5981) projected
  line L540 (-88.7253, 165.5981) -> (-85.8386, 160.5981) projected
  line L541 (-85.8386, 160.5981) -> (-88.7253, 155.5981) projected
  line L542 (-88.7253, 155.5981) -> (-94.4988, 155.5981) projected
  line L543 (-94.4988, 155.5981) -> (-97.3856, 160.5981) projected
  line L544 (-75.735, 143.0981) -> (-72.8482, 138.0981) projected
  line L545 (-72.8482, 138.0981) -> (-75.735, 133.0981) projected
  line L546 (-75.735, 133.0981) -> (-81.5085, 133.0981) projected
  line L547 (-81.5085, 133.0981) -> (-84.3952, 138.0981) projected
  line L548 (-84.3952, 138.0981) -> (-81.5085, 143.0981) projected
  line L549 (-81.5085, 143.0981) -> (-75.735, 143.0981) projected
  line L550 (-68.4988, 140.5981) -> (-71.3856, 145.5981) projected
  line L551 (-71.3856, 145.5981) -> (-68.4988, 150.5981) projected
  line L552 (-68.4988, 150.5981) -> (-62.7253, 150.5981) projected
  line L553 (-62.7253, 150.5981) -> (-59.8386, 145.5981) projected
  line L554 (-59.8386, 145.5981) -> (-62.7253, 140.5981) projected
  line L555 (-62.7253, 140.5981) -> (-68.4988, 140.5981) projected
  line L556 (-55.5085, 158.0981) -> (-49.735, 158.0981) projected
  line L557 (-49.735, 158.0981) -> (-46.8482, 153.0981) projected
  line L558 (-46.8482, 153.0981) -> (-49.735, 148.0981) projected
  line L559 (-49.735, 148.0981) -> (-55.5085, 148.0981) projected
  line L560 (-55.5085, 148.0981) -> (-58.3952, 153.0981) projected
  line L561 (-58.3952, 153.0981) -> (-55.5085, 158.0981) projected
  line L562 (-45.3856, 130.5981) -> (-42.4988, 135.5981) projected
  line L563 (-42.4988, 135.5981) -> (-36.7253, 135.5981) projected
  line L564 (-36.7253, 135.5981) -> (-33.8386, 130.5981) projected
  line L565 (-33.8386, 130.5981) -> (-36.7253, 125.5981) projected
  line L566 (-36.7253, 125.5981) -> (-42.4988, 125.5981) projected
  line L567 (-42.4988, 125.5981) -> (-45.3856, 130.5981) projected
  line L568 (-20.8482, 168.0981) -> (-23.735, 163.0981) projected
  line L569 (-23.735, 163.0981) -> (-29.5085, 163.0981) projected
  line L570 (-29.5085, 163.0981) -> (-32.3952, 168.0981) projected
  line L571 (-32.3952, 168.0981) -> (-29.5085, 173.0981) projected
  line L572 (-29.5085, 173.0981) -> (-23.735, 173.0981) projected
  line L573 (-23.735, 173.0981) -> (-20.8482, 168.0981) projected
  line L574 (-367.5102, 296.0981) -> (22.4898, 296.0981) construction
  line L575 (22.4898, 296.0981) -> (22.4898, 246.0981) construction
  line L576 (22.4898, 246.0981) -> (-367.5102, 246.0981) construction
  line L577 (-367.5102, 246.0981) -> (-367.5102, 296.0981) construction
  line L578 (-301.9111, 246.1211) -> (-308.4088, 252.6188)
  line L579 (-308.4088, 252.6188) -> (-308.4088, 296.1211)
  line L580 (-308.4088, 296.1211) -> (-290.9895, 296.1211)
  line L581 (-290.9895, 296.1211) -> (-290.9895, 246.1211)
  line L582 (-290.9895, 246.1211) -> (-301.9111, 246.1211)
  line L583 (-288.9618, 246.1211) -> (-288.9618, 260.9137)
  line L584 (-288.9618, 260.9137) -> (-256.1508, 260.9137)
  line L585 (-256.1508, 260.9137) -> (-256.1508, 246.1211)
  line L586 (-256.1508, 246.1211) -> (-288.9618, 246.1211)
  line L587 (-220.4365, 246.1672) -> (-245.3213, 246.1672)
  line L588 (-245.3213, 246.1672) -> (-253.3858, 254.2317)
  line L589 (-253.3858, 254.2317) -> (-253.3858, 282.204)
  line L590 (-253.3858, 282.204) -> (-235.736, 282.204)
  line L591 (-235.736, 282.204) -> (-235.736, 260.9598)
  line L592 (-235.736, 260.9598) -> (-220.4365, 260.9598)
  line L593 (-220.4365, 260.9598) -> (-220.4365, 246.1672)
  line L594 (-200.8512, 246.1672) -> (-218.501, 246.1672)
  line L595 (-218.501, 246.1672) -> (-218.501, 282.204)
  line L596 (-218.501, 282.204) -> (-200.8512, 282.204)
  line L597 (-200.8512, 282.204) -> (-200.8512, 246.1672)
  line L598 (-180.5286, 246.1211) -> (-191.5885, 246.1211)
  line L599 (-191.5885, 246.1211) -> (-198.0862, 252.6188)
  line L600 (-198.0862, 252.6188) -> (-198.0862, 289.6234)
  line L601 (-198.0862, 289.6234) -> (-191.5885, 296.1211)
  line L602 (-191.5885, 296.1211) -> (-180.5286, 296.1211)
  line L603 (-180.5286, 296.1211) -> (-180.5286, 246.1211)
  line L604 (-145.5517, 280.6833) -> (-178.501, 280.6833)
  line L605 (-178.501, 280.6833) -> (-178.501, 296.1211)
  line L606 (-178.501, 296.1211) -> (-145.5517, 296.1211)
  line L607 (-145.5517, 296.1211) -> (-145.5517, 280.6833)
  line L608 (-145.5517, 246.1211) -> (-178.501, 246.1211)
  line L609 (-178.501, 246.1211) -> (-178.501, 260.9137)
  line L610 (-178.501, 260.9137) -> (-145.5517, 260.9137)
  line L611 (-145.5517, 260.9137) -> (-145.5517, 246.1211)
  line L612 (-145.5517, 266.5358) -> (-178.501, 266.5358)
  line L613 (-178.501, 266.5358) -> (-178.501, 278.6557)
  line L614 (-178.501, 278.6557) -> (-145.5517, 278.6557)
  line L615 (-145.5517, 278.6557) -> (-145.5517, 266.5358)
  line L616 (-109.8374, 246.075) -> (-126.1968, 246.075)
  line L617 (-126.1968, 246.075) -> (-142.7867, 262.6649)
  line L618 (-142.7867, 262.6649) -> (-142.7867, 296.1211)
  line L619 (-142.7867, 296.1211) -> (-125.1369, 296.1211)
  line L620 (-125.1369, 296.1211) -> (-125.1369, 261.8815)
  line L621 (-125.1369, 261.8815) -> (-109.8374, 261.8815)
  line L622 (-109.8374, 261.8815) -> (-109.8374, 246.075)
  line L623 (-107.9019, 246.1211) -> (-107.9019, 296.1211)
  line L624 (-107.9019, 296.1211) -> (-90.5286, 296.1211)
  line L625 (-90.5286, 296.1211) -> (-90.5286, 262.757)
  line L626 (-90.5286, 262.757) -> (-107.9019, 246.1211)
  line L627 (-70.1139, 246.1211) -> (-81.266, 246.1211)
  line L628 (-81.266, 246.1211) -> (-87.7637, 252.6188)
  line L629 (-87.7637, 252.6188) -> (-87.7637, 289.6234)
  line L630 (-87.7637, 289.6234) -> (-81.2199, 296.1211)
  line L631 (-81.2199, 296.1211) -> (-54.8144, 296.1211)
  line L632 (-54.8144, 296.1211) -> (-54.8144, 280.6833)
  line L633 (-54.8144, 280.6833) -> (-70.1139, 280.6833)
  line L634 (-70.1139, 280.6833) -> (-70.1139, 246.1211)
  line L635 (-35.2291, 252.6649) -> (-41.7729, 246.1211)
  line L636 (-41.7729, 246.1211) -> (-68.2706, 246.1211)
  line L637 (-68.2706, 246.1211) -> (-68.2706, 260.9137)
  line L638 (-68.2706, 260.9137) -> (-52.8789, 260.9137)
  line L639 (-52.8789, 260.9137) -> (-52.8789, 296.1211)
  line L640 (-52.8789, 296.1211) -> (-41.7729, 296.1211)
  line L641 (-41.7729, 296.1211) -> (-35.2291, 289.5773)
  line L642 (-35.2291, 289.5773) -> (-35.2291, 252.6649)
  point P0 (0, 0)
  dimension "d2" = 150
  dimension "d3" = 50
  constraints: 2 vertical alignment, 2 other
  measures "d2" distance between parallel lines of L3 L576
  measures "d3" distance between parallel lines of L574 L576
extrude "Extrusion2" cut sketch "Sketch2" against normal through all contours L578 L579 L580 L581 L582 | L583 L584 L585 L586 | L587 L588 L589 L590 L591 L592 L593 | L594 L595 L596 L597 | L598 L599 L600 L601 L602 L603 | L604 L605 L606 L607 | L608 L609 L610 L611 | L612 L613 L614 L615 | L616 L617 L618 L619 L620 L621 L622 | L623 L624 L625 L626 | L627 L628 L629 L630 L631 L632 L633 L634 | L635 L636 L637 L638 L639 L640 L641 L642